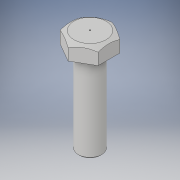
# Autodesk Inventor part: Part4
Saved by Autodesk Inventor 2019 (Build 230136000, 136)
## iProperties
Created: 2022-01-28
Part Number: Part4
Material: Generic
Document SubType Name: Modeling
Designer: Sepehr
Density: 1 g/cm^3
Appearance: Default
Author: Sepehr
Autodesk Inventor part; units mm, degrees
ref_plane "YZ Plane" through (0, 0, 0) normal (1, 0, 0) x (0, 1, 0)
ref_plane "XZ Plane" through (0, 0, 0) normal (0, 1, 0) x (-1, 0, 0)
sketch "Sketch1" plane through (0, 0, 0) normal (0, 1, 0) x (-1, 0, 0)
  line L0 (325, -187.6388) -> (0, -375.2777)
  line L1 (0, -375.2777) -> (-325, -187.6388)
  line L2 (-325, -187.6388) -> (-325, 187.6388)
  line L3 (-325, 187.6388) -> (0, 375.2777)
  line L4 (0, 375.2777) -> (325, 187.6388)
  line L5 (325, 187.6388) -> (325, -187.6388)
  point P0 (0, 0)
  point P1 (0, 0)
  point P2 (325, 0)
  constraints: 12 end point, 1 coincident, 1 midpoint, 13 other
extrude "Extrusion1" add sketch "Sketch1" against normal blind 265
sketch "Sketch2" plane through (0, -265, 0) normal (0, -1, 0) x (1, 0, 0)
  circle A0 centre (0, 0) radius 200
  dimension "d4" = 400
  constraints: 1 centre point, 1 coincident
  measures "d4" diameter of A0
extrude "Extrusion2" add sketch "Sketch2" along normal blind 1500
chamfer "Chamfer1" distance 25 angle 45 1 edges at (-200, -1765, 0)
ref_plane "Work Plane1" through (0, 0, 0) normal (0, 0, 1) x (1, 0, 0)
sketch "Sketch3" plane through (0, 0, 0) normal (0, 0, 1) x (1, 0, 0)
  point P0 (0, 0)
sketch "Sketch4" plane through (0, 0, 0) normal (0, 0, 1) x (1, 0, 0)
  line L0 (0, 0) -> (275, 0)
  line L1 (0, 0) -> (325, 0) projected
  line L2 (275, 0) -> (497.8484, -144.7195)
  line L3 (275, 0) -> (540.7163, 0) construction
  line L4 (497.8484, -144.7195) -> (497.8484, 0)
  line L5 (497.8484, 0) -> (275, 0)
  line L6 (0, -2118) -> (0, 353) projected
  dimension "d11" = 275
  dimension "d12" = 33
  constraints: 10 end point, 1 collinear, 1 equal length, 1 horizontal, 1 point on line, 1 vertical
  measures "d11" distance of L0.start L0.end
  measures "d12" angle of L2 L3
revolve "Revolution1" cut sketch "Sketch4" angle 360 about axis through (0, -10, 0) along (0, 1, 0)
body "Solid1"
